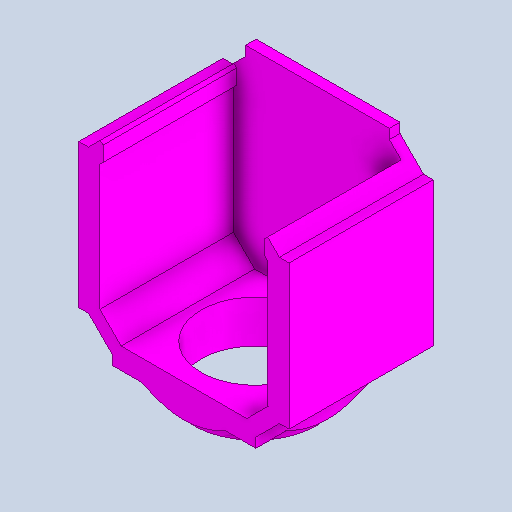
# Autodesk Inventor part: Camera Mount Side
Saved by Autodesk Inventor 2023.1 (Build 271208000, 208)
## iProperties
Created: 2022-08-10
Part Number: Camera Mount Side
Material: Generic
Document SubType Name: Modeling
Designer: xSibe
Density: 1 g/cm^3
Appearance: Plastic Magenta
Author: xSibe
Autodesk Inventor part; units mm, degrees
ref_plane "YZ Plane" through (0, 0, 0) normal (1, 0, 0) x (0, 1, 0)
ref_plane "XZ Plane" through (0, 0, 0) normal (0, 1, 0) x (-1, 0, 0)
sketch "Sketch1" plane through (0, 0, 0) normal (0, 0, 1) x (1, 0, 0)
  circle A0 centre (-10, 20.9) radius 1.875 projected
  circle A1 centre (-10, -20.9) radius 1.875 projected
  circle A2 centre (10, 20.9) radius 1.875 projected
  circle A3 centre (10, -20.9) radius 1.875 projected
  circle A4 centre (20.8, -14.4) radius 2.075 projected
  circle A5 centre (20.8, 14.4) radius 2.075 projected
  circle A6 centre (-20.8, 14.4) radius 2.075 projected
  circle A7 centre (-20.8, -14.4) radius 2.075 projected
  line L0 (16.9, -16.9) -> (-16.9, -16.9) projected
  line L1 (-16.9, -16.9) -> (-16.9, 16.9) projected
  line L2 (-16.9, 16.9) -> (16.9, 16.9) projected
  line L3 (16.9, 16.9) -> (16.9, -16.9) projected
  line L4 (-17.05, 24.9) -> (-17.05, 22.55) projected
  line L5 (-17.05, 22.55) -> (-22.55, 17.05) projected
  line L6 (-22.55, 17.05) -> (-24.9, 17.05) projected
  line L7 (-24.9, 17.05) -> (-24.9, -17.05) projected
  line L8 (-24.9, -17.05) -> (-22.55, -17.05) projected
  line L9 (-22.55, -17.05) -> (-17.05, -22.55) projected
  line L10 (-17.05, -22.55) -> (-17.05, -24.9) projected
  line L11 (-17.05, -24.9) -> (17.05, -24.9) projected
  line L12 (17.05, -24.9) -> (17.05, -22.55) projected
  line L13 (17.05, -22.55) -> (22.55, -17.05) projected
  line L14 (22.55, -17.05) -> (24.9, -17.05) projected
  line L15 (24.9, -17.05) -> (24.9, 17.05) projected
  line L16 (24.9, 17.05) -> (22.55, 17.05) projected
  line L17 (22.55, 17.05) -> (17.05, 22.55) projected
  line L18 (17.05, 22.55) -> (17.05, 24.9) projected
  line L19 (17.05, 24.9) -> (-17.05, 24.9) projected
  line L20 (24.825, 16.975) -> (24.825, -16.975)
  line L21 (24.825, -16.975) -> (22.5189, -16.975)
  line L22 (22.5189, -16.975) -> (16.975, -22.5189)
  line L23 (16.975, -22.5189) -> (16.975, -24.825)
  line L24 (16.975, -24.825) -> (-16.975, -24.825)
  line L25 (-16.975, -24.825) -> (-16.975, -22.5189)
  line L26 (-16.975, -22.5189) -> (-22.5189, -16.975)
  line L27 (-22.5189, -16.975) -> (-24.825, -16.975)
  line L28 (-24.825, -16.975) -> (-24.825, 16.975)
  line L29 (-24.825, 16.975) -> (-22.5189, 16.975)
  line L30 (-22.5189, 16.975) -> (-16.975, 22.5189)
  line L31 (-16.975, 22.5189) -> (-16.975, 24.825)
  line L32 (-16.975, 24.825) -> (16.975, 24.825)
  line L33 (16.975, 24.825) -> (16.975, 22.5189)
  line L34 (16.975, 22.5189) -> (22.5189, 16.975)
  line L35 (22.5189, 16.975) -> (24.825, 16.975)
  point P0 (0, 0)
  dimension "d0" = 0.075
  constraints: 32 end point, 15 other
  measures "d0" distance between parallel lines of L15 L20
ref_plane "Work Plane1" through (-24.9, -24.9, 7.7) normal (0, 0, 1) x (1, 0, 0)
extrude "Extrusion1" add sketch "Sketch1" along normal blind 2.5 from surface at 7.7 contours A0 | A1 | A2 | A3 | A4 | A5 | A6 | A7 | L0 L1 L2 L3 | L20 L21 L22 L23 L24 L25 L26 L27 L28 L29 L30 L31 L32 L33 L34 L35
sketch "Sketch2" plane through (0, 0, 0) normal (0, 0, 1) x (1, 0, 0)
  line L0 (22.5189, 16.975) -> (24.825, 16.975) projected
  line L1 (16.975, 22.5189) -> (22.5189, 16.975) projected
  line L2 (16.975, 24.825) -> (16.975, 22.5189) projected
  line L3 (-16.975, 24.825) -> (16.975, 24.825) projected
  line L4 (-16.975, 22.5189) -> (-16.975, 24.825) projected
  line L5 (-22.5189, 16.975) -> (-16.975, 22.5189) projected
  line L6 (-24.825, 16.975) -> (-22.5189, 16.975) projected
  line L7 (-24.825, -16.975) -> (-24.825, 16.975) projected
  line L8 (-22.5189, -16.975) -> (-24.825, -16.975) projected
  line L9 (-16.975, -22.5189) -> (-22.5189, -16.975) projected
  line L10 (-16.975, -24.825) -> (-16.975, -22.5189) projected
  line L11 (16.975, -24.825) -> (-16.975, -24.825) projected
  line L12 (16.975, -22.5189) -> (16.975, -24.825) projected
  line L13 (22.5189, -16.975) -> (16.975, -22.5189) projected
  line L14 (24.825, -16.975) -> (22.5189, -16.975) projected
  line L15 (24.825, 16.975) -> (24.825, -16.975) projected
  line L16 (24.825, -16.975) -> (24.825, -24.825)
  line L17 (24.825, -24.825) -> (16.975, -24.825)
  line L18 (24.825, -24.825) -> (14.825, -24.825)
  line L19 (14.825, -24.825) -> (14.825, -19.825)
  line L20 (19.825, -14.825) -> (24.825, -14.825)
  line L21 (24.825, -14.825) -> (24.825, -24.825)
  line L22 (19.825, -14.825) -> (14.825, -19.825)
  line L23 (14.825, 19.825) -> (19.825, 14.825)
  line L24 (14.825, 19.825) -> (14.825, 24.825)
  line L25 (14.825, 24.825) -> (24.825, 24.825)
  line L26 (24.825, 24.825) -> (24.825, 14.825)
  line L27 (24.825, 14.825) -> (19.825, 14.825)
  line L28 (-19.825, 14.825) -> (-14.825, 19.825)
  line L29 (-19.825, 14.825) -> (-24.825, 14.825)
  line L30 (-24.825, 14.825) -> (-24.825, 24.825)
  line L31 (-24.825, 24.825) -> (-14.825, 24.825)
  line L32 (-14.825, 24.825) -> (-14.825, 19.825)
  line L33 (-14.825, -19.825) -> (-19.825, -14.825)
  line L34 (-14.825, -19.825) -> (-14.825, -24.825)
  line L35 (-14.825, -24.825) -> (-24.825, -24.825)
  line L36 (-24.825, -24.825) -> (-24.825, -14.825)
  line L37 (-24.825, -14.825) -> (-19.825, -14.825)
  line L38 (16.9, -16.9) -> (19.747, -19.747)
  line L39 (-16.9, -16.9) -> (-19.747, -19.747)
  circle A0 centre (20.8, -14.4) radius 2.075 projected
  circle A1 centre (20.8, 14.4) radius 2.075 projected
  circle A2 centre (-20.8, 14.4) radius 2.075 projected
  circle A3 centre (-20.8, -14.4) radius 2.075 projected
  line L40 (16.9, -16.9) -> (-16.9, -16.9) projected
  line L41 (16.9, 16.9) -> (16.9, -16.9) projected
  line L42 (-16.9, 16.9) -> (16.9, 16.9) projected
  line L43 (-16.9, -16.9) -> (-16.9, 16.9) projected
  line L44 (24.875, -22.9) -> (24.875, 22.9) projected
  arc A4 (22.9, -24.875) -> (24.875, -22.9) centre (22.9, -22.9) ccw projected
  line L45 (-22.9, -24.875) -> (22.9, -24.875) projected
  arc A5 (-24.875, -22.9) -> (-22.9, -24.875) centre (-22.9, -22.9) ccw projected
  line L46 (-24.875, 22.9) -> (-24.875, -22.9) projected
  arc A6 (-22.9, 24.875) -> (-24.875, 22.9) centre (-22.9, 22.9) ccw projected
  line L47 (22.9, 24.875) -> (-22.9, 24.875) projected
  arc A7 (24.875, 22.9) -> (22.9, 24.875) centre (22.9, 22.9) ccw projected
  line L48 (16.9, 16.9) -> (19.747, 19.747)
  line L49 (-16.9, 16.9) -> (-19.747, 19.747)
  line L50 (14.825, -19.825) -> (-14.825, -19.825)
  line L51 (19.825, -14.825) -> (19.825, 14.825)
  line L52 (-19.825, -14.825) -> (-19.825, 14.825)
  point P0 (0, 0)
  point P1 (14.825, -14.825)
  point P2 (17.325, -17.325)
  point P3 (-17.325, -17.325)
  point P4 (24.15, -14.825)
  point P5 (22.831, -14.825)
  point P6 (19.0838, -15.5662)
  point P7 (-19.0838, -15.5662)
  point P8 (-22.831, -14.825)
  point P9 (-24.15, -14.825)
  point P10 (-24.15, 14.825)
  point P11 (-22.831, 14.825)
  point P12 (-19.0838, 15.5662)
  point P13 (-14.825, 24.15)
  point P14 (14.825, 24.15)
  point P15 (19.0838, 15.5662)
  point P16 (22.831, 14.825)
  point P17 (24.15, 14.825)
  point P18 (-17.325, 17.325)
  point P19 (17.325, 17.325)
  point P20 (-23.3416, 24.825)
  point P21 (23.3416, 24.825)
  point P22 (-24.825, -23.3416)
  point P23 (-24.825, 23.3416)
  point P24 (23.3416, -24.825)
  point P25 (-23.3416, -24.825)
  point P26 (24.825, -23.3416)
  point P27 (24.825, 23.3416)
  dimension "d3" = 10
  dimension "d4" = 10
  dimension "d5" = 5
  dimension "d6" = 5
  dimension "d9" = 360
  constraints: 58 end point, 4 midpoint, 3 parallel, 2 perpendicular, 2 point on line, 1 horizontal, 1 vertical, 41 other
  measures "d3" distance of point (14.825, -14.825) L20.end
  measures "d4" distance of L18.end point (14.825, -14.825)
  measures "d5" distance of L20.start point (14.825, -14.825)
  measures "d6" distance of L19.end point (14.825, -14.825)
extrude "Extrusion2" add sketch "Sketch2" along normal blind 31.5 from surface at 10.2 contours L0 L15 L27 A1 L23 L48 L1 | L15 L20 A0 L51 A1 L27 | L15 L14 L13 L38 L22 A0 L20 | A1 L51 L27 | L27 L23 A1 | A0 L22 L20 | L20 L51 A0 | L38 L13 L12 L11 L19 L22 | L28 A2 L29 L7 L6 L5 L49 | L19 L11 L34 L50 | L39 L9 L8 L7 L37 A3 L33 | L33 L34 L11 L10 L9 L39 | L28 L29 A2 | A3 L37 L33 | L52 A2 L29 | A2 L52 A3 L37 L7 L29 | L37 A3 L52
chamfer "Chamfer1" distance 2.5 angle 45 2 edges at (17.325, 17.325, 25.95) (-17.325, 17.325, 25.95)
sketch "Sketch3" plane through (-16.975, -24.825, 7.7) normal (0, -1, 0) x (1, 0, 0)
  line L0 (-0.075, 0) -> (-0.075, 34.4) projected
  line L1 (34.025, 0) -> (34.025, 34.4) projected
  line L2 (-0.075, 17.2) -> (34.025, 17.2)
  circle A0 centre (16.975, 17.2) radius 12.75
  point P0 (16.975, -7.7)
  dimension "d16" = 25.5
  constraints: 3 midpoint, 2 end point, 1 centre point
  measures "d16" diameter of A0
extrude "Extrusion3" cut sketch "Sketch3" against normal up to surface (5 mm away)
sketch "Sketch4" plane through (-16.975, -24.825, 7.7) normal (0, -1, 0) x (1, 0, 0)
  line L0 (33.95, 34) -> (0, 34) projected
  line L1 (0, 0) -> (0, 34) projected
  line L2 (33.95, 0) -> (0, 0) projected
  line L3 (33.95, 0) -> (33.95, 34) projected
  circle A0 centre (16.975, 17.2) radius 14.5
  circle A1 centre (16.975, 17.2) radius 12.75 projected
  point P0 (16.975, -7.7)
  dimension "d25" = 1.75
  constraints: 1 centre point, 1 coincident
  measures "d25" radial gap between concentric circles of A0 A1
extrude "Extrusion4" add sketch "Sketch4" along normal blind 5 contours A0
chamfer "Chamfer2" distance 5 angle 45 1 edges at (-14.5, -24.825, 24.9)
equation "\"d6\" = d5"
body "Solid1"
